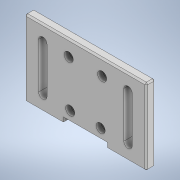
# Autodesk Inventor part: MountingAdapter
Saved by Autodesk Inventor 2020 (Build 240168000, 168)
## iProperties
Created: 2019-11-07
Part Number: MountingAdapter
Material: Generic
Document SubType Name: Modeling
Designer: nicoc
Density: 1 g/cm^3
Appearance: Default
Author: nicoc
Autodesk Inventor part; units mm, degrees
ref_plane "YZ Plane" through (0, 0, 0) normal (1, 0, 0) x (0, 1, 0)
ref_plane "XZ Plane" through (0, 0, 0) normal (0, 1, 0) x (-1, 0, 0)
ref_plane "XY Plane" through (0, 0, 0) normal (0, 0, 1) x (1, 0, 0)
sketch "Sketch1" plane through (0, 0, 0) normal (0, 0, 1) x (1, 0, 0)
  line L0 (0, 0) -> (80, 0)
  line L1 (80, 0) -> (80, 50)
  line L2 (80, 50) -> (0, 50)
  line L3 (0, 50) -> (0, 0)
  line L4 (12, 40) -> (12, 10) construction
  line L5 (9.25, 40) -> (9.25, 10)
  line L6 (14.75, 10) -> (14.75, 40)
  arc A0 (14.75, 40) -> (9.25, 40) centre (12, 40) ccw
  arc A1 (9.25, 10) -> (14.75, 10) centre (12, 10) ccw
  line L7 (68, 40) -> (68, 10) construction
  line L8 (65.25, 40) -> (65.25, 10)
  line L9 (70.75, 10) -> (70.75, 40)
  arc A2 (70.75, 40) -> (65.25, 40) centre (68, 40) ccw
  arc A3 (65.25, 10) -> (70.75, 10) centre (68, 10) ccw
  point P0 (12, 25)
  point P1 (68, 25)
  dimension "d0" = 80
  dimension "d1" = 50
  dimension "d2" = 5.5
  dimension "d3" = 12
  dimension "d5" = 30
  dimension "d6" = 12
  dimension "d8" = 5.5
  dimension "d9" = 30
  dimension "d38" = 25
  dimension "d39" = 25
  constraints: 24 end point, 8 point on circle, 8 tangent, 4 centre point, 4 parallel, 2 midpoint, 2 vertical, 1 horizontal, 1 perpendicular
  measures "d0" distance between parallel lines of L1 L3
  measures "d1" distance between parallel lines of L0 L2
  measures "d2" distance between parallel lines of L6 L5
  measures "d3" distance between parallel lines of L4 L3
  measures "d5" distance of L6.end L6.start
  measures "d6" distance between parallel lines of L7 L1
  measures "d8" distance between parallel lines of L9 L8
  measures "d9" distance of L8.start L8.end
  measures "d38" distance from line of L2 point (12, 25)
  measures "d39" distance from line of L2 point (68, 25)
extrude "Extrusion1" add sketch "Sketch1" against normal blind 6
sketch "Sketch2" plane through (0, 0, 0) normal (0, 0, 1) x (1, 0, 0)
  line L0 (0, 0) -> (80, 0) projected
  line L1 (0, 50) -> (0, 0) projected
  line L2 (0, 50) -> (80, 50) projected
  point P0 (30, 9.8)
  point P1 (29, 39.8)
  point P2 (51, 39.8)
  point P3 (50, 9.8)
  dimension "d46" = 29
  dimension "d47" = 22
  dimension "d48" = 30
  dimension "d49" = 20
  dimension "d50" = 30
  dimension "d51" = 30
  dimension "d52" = 10.2
  dimension "d53" = 10.2
  measures "d46" distance from line of point (29, 39.8) L1
  measures "d47" distance of point (51, 39.8) point (29, 39.8)
  measures "d48" distance from line of L1 point (30, 9.8)
  measures "d49" distance of point (50, 9.8) point (30, 9.8)
  measures "d50" vertical distance of point (30, 9.8) point (29, 39.8)
  measures "d51" vertical distance of point (50, 9.8) point (51, 39.8)
  measures "d52" distance from line of L2 point (29, 39.8)
  measures "d53" distance from line of L2 point (51, 39.8)
hole "Hole1" at (30, 9.8, 0) at (29, 39.8, 0) at (51, 39.8, 0) at (50, 9.8, 0) direction (0, 0, -1) diameter 3.4 end through all counterbore diameter 6 counterbore depth 3.34
sketch "Sketch4" plane through (0, 0, 0) normal (0, 0, 1) x (1, 0, 0)
  line L0 (1, 0) -> (79, 0) projected
  line L1 (54.5, 0) -> (25.5, 0)
  line L2 (25.5, 0) -> (25.5, 3)
  line L3 (25.5, 3) -> (54.5, 3)
  line L4 (54.5, 3) -> (54.5, 0)
  line L5 (80, 1) -> (80, 49) projected
  point P0 (0, 0)
  dimension "d54" = 3
  dimension "d55" = 25.5
  dimension "d56" = 29
  constraints: 8 end point, 2 parallel, 1 horizontal, 1 perpendicular, 1 point on line
  measures "d54" distance between parallel lines of L3 L0
  measures "d55" distance between parallel lines of L4 L5
  measures "d56" distance between parallel lines of L2 L4
extrude "Extrusion2" cut sketch "Sketch4" against normal through all
chamfer "Chamfer2" distance 1 angle 45 20 edges at (67.25, 0, -6) (40, 3, -6) (40, 3, 0) (54.5, 1.5, -6) (67.25, 0, 0) (54.5, 0, -3) (12.75, 0, 0) (12.75, 0, -6) (25.5, 1.5, -6) (25.5, 0, -3) (0, 25, -6) (40, 50, -6) (80, 25, -6) (80, 0, -3) (0, 0, -3) (0, 50, -3) (40, 50, 0) (0, 25, 0) (80, 50, -3) (80, 25, 0)
equation "\"d53\" = d52"
body "Solid1"
